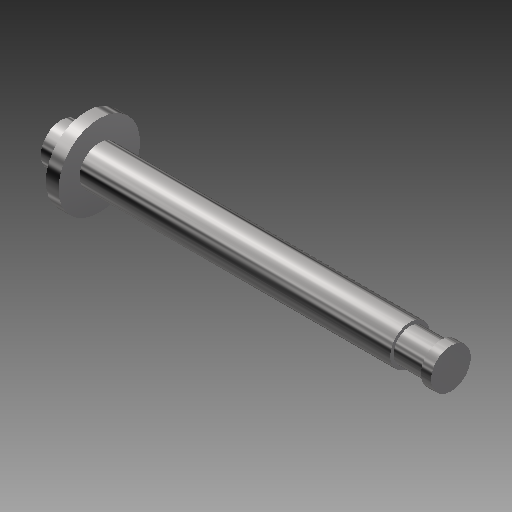
# Autodesk Inventor part: 403-06
Saved by Autodesk Inventor 2019 (Build 230136000, 136)
## iProperties
Company: Autodesk Inc.
Created: 2017-06-27
Part Number: 403-06
Material: Steel, Mild
Document SubType Name: Modeling
Designer: Autodesk Inc.
Mass: 3.88913 g
Surface Area: 5.87238 cm^2
Volume: 0.495431 cm^3
Density: 7.85 g/cm^3
Appearance: Semi-Polished
Author: Inventor
Autodesk Inventor part; units mm, degrees
ref_plane "YZ Plane" through (0, 0, 0) normal (1, 0, 0) x (0, 1, 0)
ref_plane "XZ Plane" through (0, 0, 0) normal (0, 1, 0) x (-1, 0, 0)
ref_plane "XY Plane" through (0, 0, 0) normal (0, 0, 1) x (1, 0, 0)
sketch "Sketch1" plane through (0, 0, 0) normal (0, 0, 1) x (1, 0, 0)
  line L0 (0, 0) -> (2.5, 0)
  line L1 (2.5, 0) -> (2.5, 2)
  line L2 (2.5, 2) -> (0, 2)
  line L3 (0, 2) -> (0, 0)
  line L4 (2.5, 0) -> (3.75, 0)
  line L5 (3.75, 0) -> (3.75, 4)
  line L6 (3.75, 4) -> (2.5, 4)
  line L7 (2.5, 4) -> (2.5, 0)
  line L8 (3.75, 0) -> (34.25, 0)
  line L9 (34.25, 0) -> (34.25, 1.95)
  line L10 (34.25, 1.95) -> (3.75, 1.95)
  line L11 (3.75, 1.95) -> (3.75, 0)
  line L12 (34.25, 0) -> (37.25, 0)
  line L13 (37.25, 0) -> (37.25, 1.625)
  line L14 (37.25, 1.625) -> (34.25, 1.625)
  line L15 (34.25, 1.625) -> (34.25, 0)
  line L16 (37.25, 0) -> (38.25, 0)
  line L17 (38.25, 0) -> (38.25, 1.95)
  line L18 (38.25, 1.95) -> (37.25, 1.95)
  line L19 (37.25, 1.95) -> (37.25, 0)
  dimension "d0" = 4
  dimension "d1" = 8
  dimension "d2" = 3.9
  dimension "d3" = 3.25
  dimension "d4" = 2.5
  dimension "d5" = 3.75
  dimension "d6" = 34.25
  dimension "d7" = 37.25
  dimension "d8" = 38.25
  constraints: 40 end point, 10 parallel, 5 horizontal, 5 perpendicular, 1 collinear
  measures "d0" diameter of L2 L0
  measures "d1" diameter of L6 L0
  measures "d2" diameter of L18 L16
  measures "d3" diameter of L14 L16
  measures "d4" distance of L1.end L2.end
  measures "d5" distance between parallel lines of L5 L3
  measures "d6" distance between parallel lines of L9 L3
  measures "d7" distance between parallel lines of L19 L3
  measures "d8" distance between parallel lines of L3 L17
revolve "Revolution1" add sketch "Sketch1" angle 360 about axis through (3.75, 0, 0) along (1, 0, 0)
body "Solid1"
